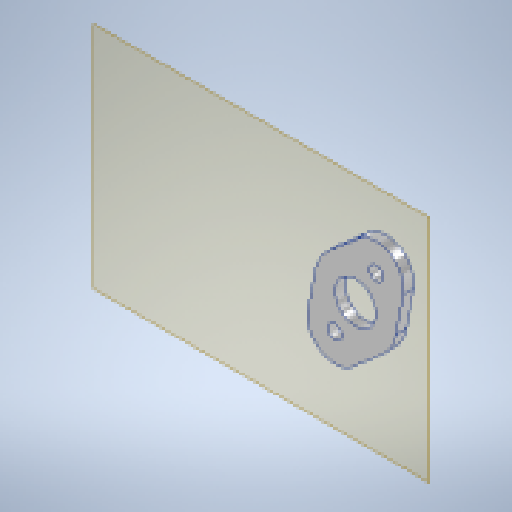
# Autodesk Inventor part: IntakeBearingBlock
Saved by Autodesk Inventor 2023 (Build 270158000, 158)
## iProperties
Created: 2022-11-10
Part Number: IntakeBearingBlock
Material: Aluminum 6061
Document SubType Name: Modeling
Designer: Zac Hah
Density: 2.7 g/cm^3
Appearance: Aluminum - Flat
Author: Zac Hah
Autodesk Inventor part; units mm, degrees
ref_plane "YZ Plane" through (0, 0, 0) normal (1, 0, 0) x (0, 1, 0)
ref_plane "XZ Plane" through (0, 0, 0) normal (0, 1, 0) x (-1, 0, 0)
ref_plane "XY Plane" through (0, 0, 0) normal (0, 0, 1) x (1, 0, 0)
ref_plane "Work Plane1" through (0, 0, 0) normal (0, 0, 1) x (1, 0, 0)
sketch "Sketch1" plane through (0, 0, 0) normal (0, 0, 1) x (1, 0, 0)
  line L0 (44.7498, 2.1658) -> (46.9612, 13.9487) projected
  arc A0 (46.9612, 13.9487) -> (42.8396, 22.8948) centre (38.5982, 15.5182) ccw projected
  arc A1 (42.8396, 22.8948) -> (22.886, 31.7216) centre (-8.8802, -67.0551) ccw projected
  arc A2 (22.886, 31.7216) -> (13.5715, 28.8544) centre (20.2809, 23.6211) ccw projected
  arc A3 (0.8003, 20.1348) -> (13.5715, 28.8544) centre (-6.4566, 44.4761) ccw projected
  line L1 (0.8003, 20.1348) -> (-28.9641, 11.2611) projected
  arc A4 (-28.9641, 11.2611) -> (-47.1072, -13.0801) centre (-21.7072, -13.0801) ccw projected
  line L2 (-47.1072, -13.0801) -> (-47.1072, -25.7801) projected
  arc A5 (-47.1072, -25.7801) -> (-40.7572, -32.1301) centre (-40.7572, -25.7801) ccw projected
  line L3 (-40.7572, -32.1301) -> (-28.0572, -32.1301) projected
  arc A6 (-28.0572, -32.1301) -> (-21.7072, -25.7801) centre (-28.0572, -25.7801) ccw projected
  line L4 (-21.7072, -25.7801) -> (-21.7072, -17.8132) projected
  arc A7 (-17.1714, -11.7279) -> (-21.7072, -17.8132) centre (-15.3572, -17.8132) ccw projected
  line L5 (-17.1714, -11.7279) -> (-5.7048, -8.3094) projected
  arc A8 (9.7562, -8.6121) -> (-5.7048, -8.3094) centre (1.552, -32.6506) ccw projected
  arc A9 (9.7562, -8.6121) -> (9.8996, -8.6596) centre (12.5046, -0.5592) ccw projected
  arc A10 (21.6959, -13.8779) -> (9.8996, -8.6596) centre (-8.8802, -67.0551) ccw projected
  arc A11 (21.6959, -13.8779) -> (31.501, -12.9394) centre (25.9373, -6.5014) ccw projected
  line L6 (31.501, -12.9394) -> (40.5717, -5.1006) projected
  arc A12 (40.5717, -5.1006) -> (44.7498, 2.1658) centre (32.2678, 4.5084) ccw projected
  arc A13 (29.1025, -0.9965) -> (35.433, 10.0133) centre (32.2678, 4.5084) ccw projected
  arc A14 (29.1025, -0.9965) -> (14.4487, 5.4859) centre (-8.8802, -67.0551) ccw construction
  arc A15 (18.3368, 17.5761) -> (14.4487, 5.4859) centre (16.3928, 11.531) ccw projected
  arc A16 (35.433, 10.0133) -> (18.3368, 17.5761) centre (-8.8802, -67.0551) ccw construction
  arc A17 (24.8611, -8.373) -> (11.8436, -2.6145) centre (-8.8802, -67.0551) ccw construction
  arc A18 (13.1656, 1.4961) -> (11.8436, -2.6145) centre (12.5046, -0.5592) ccw projected
  arc A19 (27.0135, -4.6297) -> (13.1656, 1.4961) centre (-8.8802, -67.0551) ccw construction
  arc A20 (24.8611, -8.373) -> (27.0135, -4.6297) centre (25.9373, -6.5014) ccw projected
  arc A21 (37.5221, 13.6465) -> (39.6744, 17.3899) centre (38.5982, 15.5182) ccw projected
  arc A22 (37.5221, 13.6465) -> (19.6199, 21.5658) centre (-8.8802, -67.0551) ccw construction
  arc A23 (20.9419, 25.6765) -> (19.6199, 21.5658) centre (20.2809, 23.6211) ccw projected
  arc A24 (39.6744, 17.3899) -> (20.9419, 25.6765) centre (-8.8802, -67.0551) ccw construction
  circle A25 centre (-28.0572, -25.7801) radius 2.159 projected
  circle A26 centre (-40.7572, -25.7801) radius 2.159 projected
  circle A27 centre (-40.7572, -13.0801) radius 2.159 projected
  circle A28 centre (-28.0572, -13.0801) radius 2.159 projected
  circle A29 centre (32.2678, 4.5084) radius 6.35
  circle A30 centre (25.9373, -6.5014) radius 2.159
  circle A31 centre (38.5982, 15.5182) radius 2.159
  circle A32 centre (25.9373, -6.5014) radius 8.509
  circle A33 centre (32.2678, 4.5084) radius 12.7
  circle A34 centre (38.5982, 15.5182) radius 8.509
  line L7 (23.9638, 14.1175) -> (33.0346, 21.9563)
  line L8 (19.7857, 6.851) -> (17.5743, -4.9318)
  point P0 (0, 0)
  point P1 (35.433, 10.0133)
  point P2 (29.1025, -0.9965)
  point P3 (42.8396, 22.8948)
  point P4 (21.6959, -13.8779)
  point P5 (24.8611, -8.373)
  constraints: 7 point on circle, 6 coincident, 4 centre point, 4 end point, 4 tangent, 1 concentric, 6 other
extrude "Extrusion1" add sketch "Sketch1" along normal blind 3.175 contours A33 A34 L0 | A12 A33 A32 A13 A34 | A34 A33 A21 A31 A0 | L6 A32 A33 | A34 A13 A29 A33 A31 A21 | A11 A32 A33 A30 A20 | A33 A20 A30 A32 A29 A13 | A34 A33 L7 | A29 A32 A33 A34 | L8 A33 A32
sketch "Sketch2" plane through (0, 0, 3.175) normal (0, 0, 1) x (1, 0, 0)
  circle A0 centre (32.2678, 4.5084) radius 6.35 projected
  circle A1 centre (32.2678, 4.5084) radius 5.08
  point P0 (0, 0)
  dimension "d2" = 1.27
  constraints: 1 centre point, 1 coincident
  measures "d2" radial gap between concentric circles of A0 A1
extrude "Extrusion2" add sketch "Sketch2" against normal blind 1.3716
body "Solid1"
